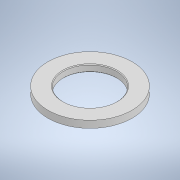
# Autodesk Inventor part: 69. Шайба упорная
Saved by Autodesk Inventor 2021 (Build 250183000, 183)
## iProperties
Created: 2021-03-11
Part Number: 69. Шайба упорная
Material: Типовые
Document SubType Name: Modeling
Designer: Данил
Density: 1 g/cm^3
Appearance: По умолчанию
Author: Данил
Autodesk Inventor part; units mm, degrees
ref_plane "YZ Plane" through (0, 0, 0) normal (1, 0, 0) x (0, 1, 0)
ref_plane "XZ Plane" through (0, 0, 0) normal (0, 1, 0) x (-1, 0, 0)
ref_plane "XY Plane" through (0, 0, 0) normal (0, 0, 1) x (1, 0, 0)
sketch "Эскиз1" plane through (0, 0, 0) normal (0, 0, 1) x (1, 0, 0)
  line L0 (0, 2.5) -> (0, -2.5)
  line L1 (19, -2) -> (19, 2)
  line L2 (19.5, 2.5) -> (30, 2.5)
  line L3 (30, 2.5) -> (30, -2.5)
  line L4 (30, -2.5) -> (19.5, -2.5)
  line L5 (19, -2) -> (19.5, -2.5)
  line L6 (19, 2) -> (19.5, 2.5)
  point P0 (0, 0)
  point P1 (0, 0)
  point P2 (19, -2.5)
  point P3 (19, 2.5)
  dimension "d0" = 5
  dimension "d1" = 60
  dimension "d2" = 38
  dimension "d3" = 0.5
  dimension "d4" = 45
  dimension "d5" = 0.5
  dimension "d6" = 45
  constraints: 14 end point, 4 point on line, 3 perpendicular, 2 horizontal alignment, 2 vertical, 1 coincident, 1 midpoint
  measures "d0" distance of L0.start L0.end
  measures "d1" diameter of L3 L0
  measures "d2" diameter of L1 L0
  measures "d3" distance of L1.start point (19, -2.5)
  measures "d4" angle of L1 L5
  measures "d5" distance of L1.end point (19, 2.5)
  measures "d6" angle of L1 L6
revolve "Вращение1" add sketch "Эскиз1" angle 360 about axis through (0, 2.5, 0) along (0, -1, 0)
